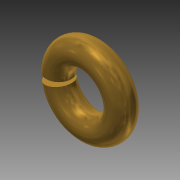
# Autodesk Inventor part: 载板连接销卡环
Saved by Autodesk Inventor 2015 (Build 190159000, 159)
## iProperties
Created: 2017-05-02
Part Number: 载板连接销卡环
Material: 常规
Document SubType Name: Modeling
Designer: Administrator
Density: 1 g/cm^3
Appearance: 黄铜 - 缎光
Author: Administrator
Autodesk Inventor part; units mm, degrees
ref_plane "YZ Plane" through (0, 0, 0) normal (1, 0, 0) x (0, 1, 0)
ref_plane "XZ Plane" through (0, 0, 0) normal (0, 1, 0) x (-1, 0, 0)
ref_plane "XY Plane" through (0, 0, 0) normal (0, 0, 1) x (1, 0, 0)
sketch "草图1" plane through (0, 0, 0) normal (0, 0, 1) x (1, 0, 0)
  circle A0 centre (-5, 0) radius 2
  line L0 (0, -2.8) -> (0, 2.8) projected
  line L1 (0, 0) -> (1.7205, 0)
  dimension "d0" = 4
  dimension "d2" = 5
  constraints: 2 end point, 1 centre point, 1 horizontal, 1 point on line
  measures "d0" diameter of A0
  measures "d2" distance of L1.start A0.centre
revolve "旋转1" add sketch "草图1" angle 350 about axis through (0, -10, 0) along (0, 1, 0)
